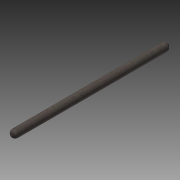
# Autodesk Inventor part: staff
Saved by Autodesk Inventor 2015 (Build 190159000, 159)
## iProperties
Created: 2015-02-05
Part Number: staff
Material: Generic
Document SubType Name: Modeling
Designer: Paul
Density: 1 g/cm^3
Appearance: Default
Author: Paul
Autodesk Inventor part; units mm, degrees
ref_plane "YZ Plane" through (0, 0, 0) normal (1, 0, 0) x (0, 1, 0)
ref_plane "XZ Plane" through (0, 0, 0) normal (0, 1, 0) x (-1, 0, 0)
ref_plane "XY Plane" through (0, 0, 0) normal (0, 0, 1) x (1, 0, 0)
sketch "Sketch1" plane through (0, 0, 0) normal (0, 0, 1) x (1, 0, 0)
  arc A0 (-0.89, 0.7514) -> (0.89, 0.7514) centre (0, -0.1263) ccw projected
  circle A1 centre (0, -0.1263) radius 1.25
  point P0 (0, 0)
  constraints: 1 coincident, 3 other
extrude "Extrusion1" add sketch "Sketch1" along normal blind 50.8
chamfer "Chamfer1" distance 1.016 angle 45 1 edges at (-1.25, -0.1263, 0)
fillet "Fillet1" radius 1.016 1 edges at (-1.25, -0.1263, 50.8)
body "Solid1"
